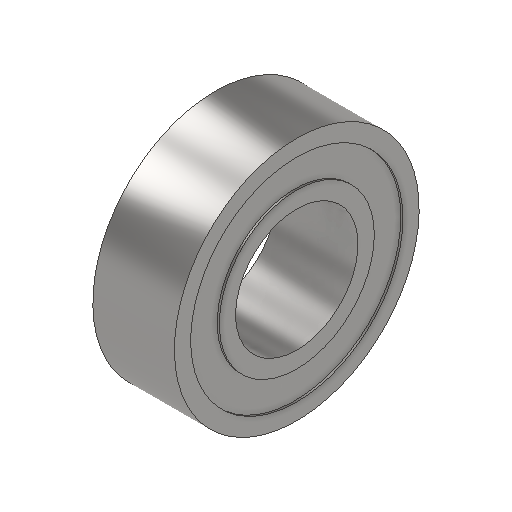
# Autodesk Inventor part: MR126ZZ-6x12x4mm
Saved by Autodesk Inventor 2025.3 (Build 293356000, 356)
## iProperties
Created: 2025-11-11
Part Number: MR126ZZ-6x12x4mm
Material: Stainless Steel
Document SubType Name: Modeling
Designer: Gabriel Bojaca
Density: 8 g/cm^3
Appearance: Semi-Polished
Author: Gabriel Bojaca
Autodesk Inventor part; units mm, degrees
ref_plane "YZ Plane" through (0, 0, 0) normal (1, 0, 0) x (0, 1, 0)
ref_plane "XZ Plane" through (0, 0, 0) normal (0, 1, 0) x (-1, 0, 0)
ref_plane "XY Plane" through (0, 0, 0) normal (0, 0, 1) x (1, 0, 0)
sketch "Sketch1" plane through (0, 0, 0) normal (1, 0, 0) x (0, 1, 0)
  circle A0 centre (0, 0) radius 6
  circle A1 centre (0, 0) radius 3
  dimension "d0" = 12
  dimension "d1" = 6
  constraints: 2 centre point, 2 coincident
  measures "d0" diameter of A0
  measures "d1" diameter of A1
extrude "Extrusion1" add sketch "Sketch1" along normal blind 4
sketch "Sketch2" plane through (0, 0, 0) normal (-1, 0, 0) x (0, 0, 1)
  circle A0 centre (0, 0) radius 6 projected
  circle A1 centre (0, 0) radius 3 projected
  circle A2 centre (0, 0) radius 5.2
  circle A3 centre (0, 0) radius 3.8
  dimension "d4" = 0.8
  dimension "d5" = 0.8
  constraints: 2 centre point
  measures "d4" radial gap between concentric circles of A0 A2
  measures "d5" radial gap between concentric circles of A1 A3
extrude "Extrusion2" cut sketch "Sketch2" against normal blind 0.1 contours A2
sketch "Sketch3" plane through (4, 0, 0) normal (1, 0, 0) x (0, 0, -1)
  circle A0 centre (0, 0) radius 6 projected
  circle A1 centre (0, 0) radius 5.2 projected
  circle A2 centre (0, 0) radius 3.8 projected
extrude "Extrusion3" cut sketch "Sketch3" against normal blind 0.1 contours A1
body "Solid1"
